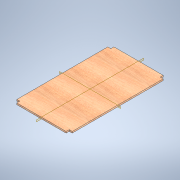
# Autodesk Inventor part: baseForLongRobot
Saved by Autodesk Inventor 2020.2 (Build 242310000, 310)
## iProperties
Created: 2020-01-09
Part Number: baseForLongRobot
Material: Wood (Birch)
Document SubType Name: Modeling
Designer: steele
Density: 0.55 g/cm^3
Appearance: Birch - Natural Polished
Author: steele
Autodesk Inventor part; units mm, degrees
ref_plane "XZ Plane" through (0, 0, 0) normal (0, 1, 0) x (-1, 0, 0)
sketch "Sketch1" plane through (0, 0, 0) normal (0, 1, 0) x (-1, 0, 0)
  line L0 (206.375, 406.4) -> (-206.375, 406.4)
  line L1 (-231.775, 381) -> (-231.775, -381)
  line L2 (-206.375, -406.4) -> (206.375, -406.4)
  line L3 (231.775, -381) -> (231.775, 381)
  line L4 (231.775, 406.4) -> (-231.775, -406.4) construction
  line L5 (-231.775, 406.4) -> (231.775, -406.4) construction
  line L6 (206.375, -406.4) -> (206.375, -381)
  line L7 (206.375, -381) -> (231.775, -381)
  line L8 (-206.375, -406.4) -> (-206.375, -381)
  line L9 (-206.375, -381) -> (-231.775, -381)
  line L10 (206.375, 406.4) -> (206.375, 381)
  line L11 (206.375, 381) -> (231.775, 381)
  line L12 (-206.375, 406.4) -> (-206.375, 381)
  line L13 (-206.375, 381) -> (-231.775, 381)
  point P0 (0, 0)
  dimension "d12" = 812.8
  dimension "d13" = 463.55
  constraints: 28 end point, 2 midpoint, 2 parallel, 1 horizontal, 1 perpendicular
  measures "d12" distance between parallel lines of L0 L2
  measures "d13" distance between parallel lines of L1 L3
extrude "Extrusion1" add sketch "Sketch1" along normal blind 12.7
body "Solid1"
